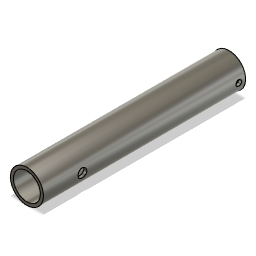
Tube 49 pour attache de bras de rappel, longueur h+20 (280+20=300mm) - VZC 21465_204505 Rep. 105 (Autodesk Fusion 360 design; units mm, degrees)
Autodesk Fusion 360 part; units mm, degrees
sketch "Sketch1" plane through (0, 0, 0) normal (0, 0, 1) x (1, 0, 0)
  circle A0 centre (0, 0) radius 24.5
  circle A1 centre (0, 0) radius 20
  dimension "d1" = 49
  dimension "d2" = 4.5
  constraint coincident A0.centre A1.centre
  measures "d1" diameter of A0
extrude "Extrude1" add sketch "Sketch1" along normal blind 300
ref_plane "WorkPlane1" through (0, 0, 10) normal (0, 0, 1) x (1, 0, 0)
ref_plane "WorkPlane2" through (0, 0, 300) normal (0, 0, 1) x (1, 0, 0)
ref_plane "WorkPlane3" through (0, 0, 242) normal (0, 0, 1) x (1, 0, 0)
sketch "Sketch2" plane through (0, 0, 0) normal (1, 0, 0) x (0, 0, -1)
  line L0 (-10, 42.4058) -> (-10, 1.4623) construction
  line L1 (-300, 66.3479) -> (-300, -66.3479) construction
  line L2 (-242, 79.6175) -> (-242, -79.6175) construction
  line L3 (-300, 0) -> (0, 0) construction
  line L4 (-10, 1.4623) -> (-10, 0) construction
  circle A0 centre (-10, 0) radius 4.25
  circle A1 centre (-242, 0) radius 6.5
  dimension "d8" = 8.5
  dimension "d9" = 13
  constraint midpoint L1 L3.start
  constraint coincident L3.end origin
  constraint coincident L0.end L4.start
  constraint coincident L3 L4.end
  constraint perpendicular L3 L4
  constraint coincident L4.end A0.centre
  constraint midpoint L2 A1.centre
  measures "d8" diameter of A0
  measures "d9" diameter of A1
extrude "Extrude2" cut sketch "Sketch2" along normal through all and the other way through all
